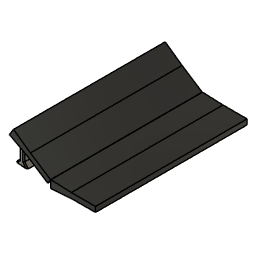
Macro Keyboards (Autodesk Fusion 360 design; units mm, degrees)
Autodesk Fusion 360 part; units mm, degrees
sketch "Sketch1" plane through (0, 0, 0) normal (1, 0, 0) x (0, 1, 0)
  line L0 (0, 0) -> (440, 0)
  line L1 (440, 0) -> (440, 22.5)
  line L2 (440, 22.5) -> (0, 22.5)
  line L3 (0, 22.5) -> (0, 0)
  dimension "d1" = 440
  dimension "d2" = 22.5
  constraint horizontal L0
  constraint vertical L1
  constraint horizontal L2
  constraint vertical L3
  constraint coincident L0.start L3.end
  measures "d1" distance of L0.start L0.end
  measures "d2" distance of L0.start L2.end
ref_plane "WorkPlane1" through (130, 220, 11.25) normal (1, 0, 0) x (0, 1, 0)
ref_plane "WorkPlane2" through (60, 0, 0) normal (1, 0, 0) x (0, 1, 0)
sketch "Sketch2" plane through (130, 0, 0) normal (1, 0, 0) x (0, 1, 0)
  line L0 (0, 0) -> (0, 5)
  line L1 (0, 5) -> (440, 5)
  line L2 (440, 5) -> (440, 20)
  line L3 (440, 20) -> (0, 20)
  line L4 (0, 20) -> (0, 5)
  dimension "d10" = 5
  dimension "d11" = 440
  dimension "d12" = 15
  constraint coincident L0.start origin
  constraint vertical L0
  constraint horizontal L1
  constraint vertical L2
  constraint horizontal L3
  constraint vertical L4
  measures "d10" distance of L0.start L0.end
  measures "d11" distance of L0.end L1.end
  measures "d12" distance of L0.end L3.end
sketch "Sketch3" plane through (60, 0, 0) normal (1, 0, 0) x (0, 1, 0)
  line L0 (0, 0) -> (0, 5)
  line L1 (0, 5) -> (440, 5)
  line L2 (440, 5) -> (440, 20)
  line L3 (440, 20) -> (0, 20)
  line L4 (0, 20) -> (0, 5)
  dimension "d7" = 5
  dimension "d8" = 440
  dimension "d9" = 15
  constraint coincident L0.start origin
  constraint vertical L0
  constraint horizontal L1
  constraint vertical L2
  constraint horizontal L3
  constraint vertical L4
  measures "d7" distance of L0.start L0.end
  measures "d8" distance of L0.end L1.end
  measures "d9" distance of L0.end L3.end
loft "Loft2" add profiles "Sketch1", "Sketch3" section 1 section 2 makes body 1
loft "Loft3" add profiles "Sketch2" section 1 face at (60, 293.3333, 15) section 2 on bodies 1 bodies 1
copy_body "CopyPasteBodies1" bodies 1 makes body 2
move_body "Move1" bodies 2 to x (0.838671, 0, -0.544639) y (0, 1, 0) z (0.544639, 0, 0.838671) at (-119.9566, 0, 75.9582)
sketch "Sketch4" plane through (0, 0, 0) normal (0, -1, 0) x (1, 0, 0)
  line L0 (-107.7023, 94.8283) -> (-119.9566, 75.9582)
  line L1 (-119.9566, 75.9582) -> (-66.9132, 47.4732)
  line L2 (-66.9132, 47.4732) -> (-8.2063, 9.3485)
  line L3 (-8.2063, 9.3485) -> (-0.0367, 21.9285)
  line L4 (-0.0367, 21.9285) -> (-58.7436, 60.0533)
  line L5 (-58.7436, 60.0533) -> (-107.7023, 94.8283)
  line L6 (-8.2063, 9.3485) -> (-16.593, 14.7949)
  line L7 (0, 0) -> (-150, 0)
  line L8 (-16.593, 14.7949) -> (-29.173, 22.9644)
  line L9 (-29.173, 22.9644) -> (-29.173, 0)
  line L10 (-16.593, 14.7949) -> (-16.593, 0)
  line L11 (-119.9566, 75.9582) -> (-111.1466, 71.2271)
  line L12 (-111.1466, 71.2271) -> (-97.9315, 64.1304)
  line L13 (-97.9315, 64.1304) -> (-97.9315, 0)
  line L14 (-111.1466, 71.2271) -> (-111.1466, 0)
  line L15 (-111.1466, 0) -> (-121.1466, 0)
  line L16 (-121.1466, 0) -> (-121.1466, 10)
  line L17 (-121.1466, 10) -> (-111.1466, 10)
  line L18 (-111.1466, 10) -> (-111.1466, 0)
  line L19 (-97.9315, 0) -> (-87.9315, 0)
  line L20 (-97.9315, 10) -> (-97.9315, 0)
  line L21 (-121.1466, 0) -> (-111.1466, 10)
  line L22 (-97.9315, 64.1304) -> (-80.3115, 54.6682)
  line L23 (-80.3115, 54.6682) -> (-80.3115, 51.6682)
  line L24 (-80.3115, 51.6682) -> (-97.9315, 51.6682)
  line L25 (-80.3115, 51.6682) -> (-97.9315, 34.0482)
  line L26 (-87.9315, 0) -> (-87.9315, -3)
  line L27 (-87.9315, -3) -> (-121.1466, 0)
  line L28 (-97.9315, 10) -> (-87.9315, -3)
  dimension "d13" = 10
  dimension "d14" = 150
  dimension "d15" = 15
  dimension "d16" = 10
  dimension "d17" = 15
  dimension "d18" = 10
  dimension "d19" = 10
  dimension "d20" = 10
  dimension "d21" = 10
  dimension "d32" = 20
  dimension "d33" = 3
  dimension "d34" = 135
  dimension "d35" = 3
  constraint coincident L2.end L3.start
  constraint perpendicular L3 L6
  constraint coincident L7.start origin
  constraint horizontal L7
  constraint parallel L2 L8
  constraint coincident L7 L9.end
  constraint perpendicular L7 L9
  constraint coincident L7 L10.end
  constraint perpendicular L7 L10
  constraint coincident L0.end L1.start
  constraint coincident L1 L11.end
  constraint coincident L1 L12.end
  constraint coincident L7 L13.end
  constraint perpendicular L7 L13
  constraint coincident L7 L14.end
  constraint perpendicular L7 L14
  constraint horizontal L15
  constraint vertical L16
  constraint horizontal L17
  constraint vertical L18
  constraint horizontal L19
  constraint vertical L20
  constraint parallel L1 L22
  constraint vertical L23
  constraint coincident L13 L24.end
  constraint perpendicular L13 L24
  constraint coincident L13 L25.end
  constraint perpendicular L19 L26
  measures "d13" distance of L2.end L6.end
  measures "d14" distance of L7.start L7.end
  measures "d15" distance of L6.end L8.end
  measures "d16" distance of L0.end L11.end
  measures "d17" distance of L11.end L12.end
  measures "d18" distance of L14.end L15.end
  measures "d19" distance of L14.end L17.end
  measures "d20" distance of L13.end L19.end
  measures "d21" distance of L13.end L20.start
  measures "d32" distance of L12.end L22.end
  measures "d33" distance of L22.end L23.end
  measures "d34" angle of L24 L25
  measures "d35" distance of L19.end L26.end
extrude "Extrude1" add sketch "Sketch4" against normal blind 60 separate body contours L1 L7 L12 L13 L14 L18 L20 | L1 L13 L22 L23 L24 | L7 L14 L15 L18 L21 | L13 L24 L25 | L7 L15 L19 L27 L28 | L7 L13 L19 L20 L28 makes body 3
extrude "Extrude2" cut 1 faces at (-92.0582, 0, 49.949) along direction (0, 1, 0) blind 20 on bodies 3 bodies 3
copy_body "CopyPasteBodies2" bodies 3 makes body 4
move_body "Move2" bodies 3 to x (1, 0, 0) y (0, 1, 0) z (0, 0, 1) at (0, 360, 0)
chamfer "Chamfer2" distance 3 angle 45 24 edges at (-111.1466, 420, 40.6135) (-97.9315, 420, 22.0241) (-116.1466, 420, 5) (-116.1466, 380, 5) (-111.1466, 380, 40.6135) (-97.9315, 380, 22.0241) (-89.1215, 420, 42.8582) (-89.1215, 380, 42.8582) (-80.3115, 380, 53.1682) (-80.3115, 420, 53.1682) (-92.9315, 420, 3.5) (-92.9315, 380, 3.5) (-97.9315, 20, 22.0241) (-116.1466, 20, 5) (-111.1466, 20, 40.6135) (-97.9315, 60, 22.0241) (-111.1466, 60, 40.6135) (-116.1466, 60, 5) (-89.1215, 20, 42.8582) (-89.1215, 60, 42.8582) (-80.3115, 20, 53.1682) (-80.3115, 60, 53.1682) (-92.9315, 20, 3.5) (-92.9315, 60, 3.5) on bodies 3 4
extrude "Extrude3" add sketch "Sketch4" against normal blind 100 separate body contours L2 L7 L8 L9 L10 makes body 5
extrude "Extrude4" cut sketch "Sketch4" against normal blind 20 contours L2 L7 L8 L9 L10 bodies 5
copy_body "CopyPasteBodies3" bodies 5 makes body 6
move_body "Move3" bodies 6 to x (1, 0, 0) y (0, 1, 0) z (0, 0, 1) at (0, 320, 0)
ref_plane "WorkPlane3" through (-22.883, 60, 22) normal (0, 0, -1) x (-1, 0, 0)
split "Split1" by plane through (-22.883, 60, 22) normal (0, 0, -1) bodies 3 4 makes body 8 at (-100.4178, 33.3333, -1.8722) makes body 7 at (-100.4178, 406.6667, -1.8722)
move_body "Move4" bodies 8 7 to x (1, 0, 0) y (0, 1, 0) z (0, 0, 1) at (0, 0, -3)
extrude "Extrude6" add 2 faces at (-102.3366, 394.3333, 22) (-102.3366, 45.6667, 22) along direction (0, 0, -1) blind 4 on bodies 3 4 bodies 3 4 7 8
extrude "Extrude7" add 2 faces at (-20.7863, 366.6667, 0) (-20.7863, 46.6667, 0) along direction (0, 0, -1) blind 3 on bodies 5 6 bodies 6 5
equation "d6 = 130 mm - 70 mm"
named bodies: "Bottom Keyboard", "Top Keyboard"
